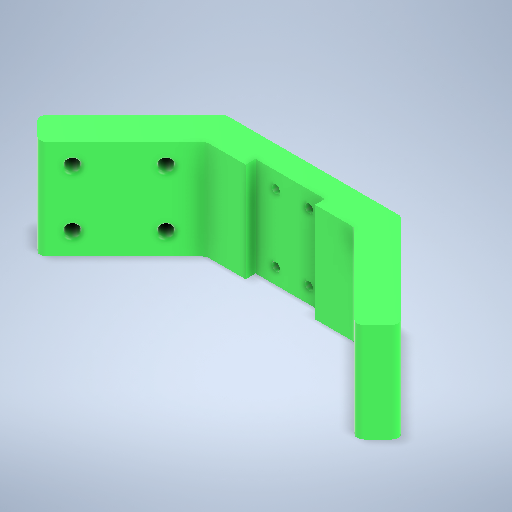
# Autodesk Inventor part: Cross Links
Saved by Autodesk Inventor 2026.2 (Build 302298010, 298A)
## iProperties
Created: 2026-03-12
Part Number: Cross Links
Material: PLA 1.75mm 50 Infill
Document SubType Name: Modeling
Designer: tngzj
Density: 0.625 g/cm^3
Appearance: PLA Plastic
Author: tngzj
Autodesk Inventor part; units mm, degrees
ref_plane "YZ Plane" through (0, 0, 0) normal (1, 0, 0) x (0, 1, 0)
ref_plane "XZ Plane" through (0, 0, 0) normal (0, 1, 0) x (-1, 0, 0)
ref_plane "XY Plane" through (0, 0, 0) normal (0, 0, 1) x (1, 0, 0)
sketch "Sketch1" plane through (0, 0, 0) normal (0, 1, 0) x (-1, 0, 0)
  line L0 (26.533, 7.0711) -> (-26.533, 7.0711) construction
  line L1 (-26.533, 7.0711) -> (-26.533, -7.0711) construction
  line L2 (-26.533, -7.0711) -> (26.533, -7.0711) construction
  line L3 (26.533, -7.0711) -> (26.533, 7.0711) construction
  line L4 (26.533, 7.0711) -> (-26.533, -7.0711) construction
  line L5 (-26.533, 7.0711) -> (26.533, -7.0711) construction
  line L6 (26.533, -7.0711) -> (55.0002, 21.3962)
  line L7 (47.9292, 28.4672) -> (55.0002, 21.3962)
  line L8 (23.9109, 2.988) -> (30.2515, -3.3526) construction
  line L9 (0, 7.0711) -> (0, -7.0711) construction
  line L10 (26.533, 7.0711) -> (22.3909, 2.9289)
  line L11 (22.3909, 2.9289) -> (0, 2.9289)
  line L12 (0, 2.9289) -> (0, -7.0711)
  line L13 (0, -7.0711) -> (22.3909, -7.0711)
  line L14 (22.3909, -7.0711) -> (22.3909, 2.9289) construction
  line L15 (26.533, -7.0711) -> (22.3909, -7.0711)
  line L16 (26.533, 7.0711) -> (47.9292, 28.4672)
  point P0 (0, 0)
  dimension "d0" = 135
  dimension "d2" = 35
  dimension "d3" = 10
  dimension "d4" = 10
  dimension "d5" = 26.533
  constraints: 34 end point, 5 perpendicular, 4 midpoint, 4 parallel, 2 collinear, 2 horizontal, 1 point on line
  measures "d0" angle of L2 L6
  measures "d2" distance from line of L7 L8.end
  measures "d3" distance of L7.start L6.end
  measures "d4" distance from line of L2 L10.end
  measures "d5" distance between parallel lines of L12 L3
extrude "Extrusion1" add sketch "Sketch1" along normal blind 30
sketch "Sketch3" plane through (-55.0002, 0, 21.3962) normal (-0.7071068, 0, -0.7071068) x (-0.7071068, 0, 0.7071068)
  line L0 (0, 0) -> (0, 30) construction
  line L1 (-40.2587, 0) -> (0, 0) construction
  line L2 (-40.2587, 30) -> (0, 30) construction
  line L3 (0, 30) -> (-35, 0) construction
  line L4 (0, 0) -> (-35, 30) construction
  line L5 (-35, 30) -> (-35, 0) construction
  line L6 (-27.5, 6.4286) -> (-7.5, 6.4286) construction
  line L7 (-7.5, 6.4286) -> (-7.5, 23.5714) construction
  line L8 (-7.5, 23.5714) -> (-27.5, 23.5714) construction
  line L9 (-27.5, 23.5714) -> (-27.5, 6.4286) construction
  line L10 (-27.5, 6.4286) -> (-7.5, 23.5714) construction
  line L11 (-7.5, 6.4286) -> (-27.5, 23.5714) construction
  circle A0 centre (-27.5, 23.5714) radius 1.8
  circle A1 centre (-7.5, 23.5714) radius 1.8
  circle A2 centre (-7.5, 6.4286) radius 1.8
  circle A3 centre (-27.5, 6.4286) radius 1.8
  point P0 (-17.5, 15)
  dimension "d15" = 35
  dimension "d16" = 20
  dimension "d17" = 3.6
  dimension "d18" = 3.6
  dimension "d19" = 3.6
  dimension "d20" = 3.6
  constraints: 18 end point, 4 centre point, 4 coincident, 3 midpoint, 3 point on line, 2 parallel, 2 perpendicular, 1 horizontal
  measures "d15" distance of L0.start L3.end
  measures "d16" distance of L7.end L8.end
  measures "d17" diameter of A0
  measures "d18" diameter of A1
  measures "d19" diameter of A3
  measures "d20" diameter of A2
extrude "Extrusion3" cut sketch "Sketch3" against normal up to surface (10 mm away)
mirror "Mirror1" about plane through (0, 0, 2.9289) normal (1, 0, 0) of "Extrusion1", "Extrusion3"
fillet "Fillet1" radius 2 8 edges at (-26.533, 15, -7.0711) (26.533, 15, -7.0711) (22.3909, 15, 2.9289) (-22.3909, 15, 2.9289) (-47.9292, 15, 28.4672) (-55.0002, 15, 21.3962) (47.9292, 15, 28.4672) (55.0002, 15, 21.3962)
fillet "Fillet3" radius 1 16 edges at (-41.3531, 23.5714, 21.8911) (-27.2109, 23.5714, 7.749) (-27.2109, 6.4286, 7.749) (-41.3531, 6.4286, 21.8911) (27.2109, 23.5714, 7.749) (41.3531, 23.5714, 21.8911) (41.3531, 6.4286, 21.8911) (27.2109, 6.4286, 7.749) (48.4241, 23.5714, 14.8201) (34.282, 23.5714, 0.6779) (34.282, 6.4286, 0.6779) (48.4241, 6.4286, 14.8201) (-34.282, 23.5714, 0.6779) (-48.4241, 23.5714, 14.8201) (-48.4241, 6.4286, 14.8201) (-34.282, 6.4286, 0.6779)
sketch "Sketch4" plane through (-21.5624, 0, 2.9289) normal (0, 0, 1) x (1, 0, 0)
  line L0 (0, 0) -> (0, 30) construction
  line L1 (0, 0) -> (43.1249, 0) construction
  line L2 (43.1249, 30) -> (43.1249, 0) construction
  line L3 (0, 30) -> (43.1249, 30) construction
  line L4 (21.5624, 0) -> (21.5624, 30) construction
  line L5 (-1.4142, 0) -> (0, 0) projected
  line L6 (0, 0) -> (43.1249, 30) construction
  line L7 (32.0624, 0) -> (11.0624, 0)
  line L8 (11.0624, 0) -> (11.0624, 30)
  line L9 (11.0624, 30) -> (32.0624, 30)
  line L10 (32.0624, 30) -> (32.0624, 0)
  line L11 (32.0624, 0) -> (11.0624, 30) construction
  line L12 (11.0624, 0) -> (32.0624, 30) construction
  point P0 (21.5624, 15)
  dimension "d26" = 21
  constraints: 16 end point, 4 midpoint, 2 parallel, 1 horizontal, 1 perpendicular, 1 point on line
  measures "d26" distance between parallel lines of L8 L10
extrude "Extrusion4" cut sketch "Sketch4" against normal blind 3
sketch "Sketch5" plane through (-21.5624, 0, -0.0711) normal (0, 0, 1) x (1, 0, 0)
  line L0 (11.0624, 30) -> (32.0624, 30) construction
  line L1 (11.0624, 0) -> (11.0624, 30) construction
  line L2 (32.0624, 0) -> (11.0624, 0) construction
  line L3 (32.0624, 30) -> (32.0624, 0) construction
  line L4 (11.0624, 30) -> (32.0624, 30) construction
  line L5 (21.5624, 30) -> (21.5624, 25.15) construction
  line L6 (11.0624, 25.15) -> (32.0624, 25.15) construction
  circle A0 centre (17.1918, 25.15) radius 1.25
  circle A1 centre (27.1848, 25.15) radius 1.25
  point P0 (21.5624, 0)
  dimension "d29" = 4.85
  dimension "d30" = 2.5
  dimension "d31" = 2.5
  dimension "d32" = 9.993
  constraints: 4 end point, 3 point on line, 2 centre point, 2 midpoint, 1 perpendicular, 1 vertical
  measures "d29" distance of L5.start L5.end
  measures "d30" diameter of A0
  measures "d31" diameter of A1
  measures "d32" distance of A1.centre A0.centre
extrude "Extrusion5" cut sketch "Sketch5" against normal up to surface (7 mm away)
ref_plane "Work Plane1" through (0, 15, 0) normal (0, 1, 0) x (1, 0, 0)
mirror "Mirror2" about plane through (0, 15, 0) normal (0, 1, 0) of "Extrusion5"
equation "\"d18\" = d17"
equation "\"d19\" = d17"
equation "\"d20\" = d17"
body "Solid1"
